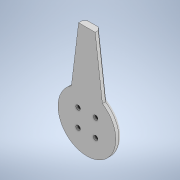
# Autodesk Inventor part: Pointerlever
Saved by Autodesk Inventor 2021 (Build 250183000, 183)
## iProperties
Created: 2024-04-28
Part Number: Pointerlever
Material: Generic
Document SubType Name: Modeling
Designer: Lukas
Density: 1 g/cm^3
Appearance: Default
Author: Lukas
Autodesk Inventor part; units mm, degrees
ref_plane "YZ Plane" through (0, 0, 0) normal (1, 0, 0) x (0, 1, 0)
ref_plane "XZ Plane" through (0, 0, 0) normal (0, 1, 0) x (-1, 0, 0)
ref_plane "XY Plane" through (0, 0, 0) normal (0, 0, 1) x (1, 0, 0)
sketch "Sketch1" plane through (0, 0, 0) normal (0, 0, 1) x (1, 0, 0)
  circle A0 centre (0, 0) radius 14
  circle A1 centre (-4.25, 4.25) radius 1.1
  circle A2 centre (-4.25, -4.25) radius 1.1
  circle A3 centre (4.25, -4.25) radius 1.1
  circle A4 centre (4.25, 4.25) radius 1.1
  line L0 (-7.5, 11.8216) -> (-4, 40)
  line L1 (-4, 40) -> (4, 40)
  line L2 (4, 40) -> (7.5, 11.8216)
  point P0 (0, 40)
  dimension "d0" = 8.5
  dimension "d1" = 8.5
  dimension "d2" = 4.25
  dimension "d3" = 4.25
  dimension "d4" = 2.2
  dimension "d5" = 28
  dimension "d6" = 8
  dimension "d7" = 15
  dimension "d8" = 40
  constraints: 6 end point, 5 centre point, 3 equal radius, 3 horizontal alignment, 3 vertical alignment, 2 point on circle, 1 coincident, 1 horizontal, 1 midpoint
  measures "d0" distance of A2.centre A1.centre
  measures "d1" distance of A3.centre A2.centre
  measures "d2" horizontal distance of point (0, 0) A2.centre
  measures "d3" horizontal distance of point (0, 0) A2.centre
  measures "d4" diameter of A1
  measures "d5" diameter of A0
  measures "d6" distance of L0.end L1.end
  measures "d7" distance of L2.end L0.start
  measures "d8" distance from line of point (0, 0) L1
extrude "Extrusion1" add sketch "Sketch1" along normal blind 1
sketch "Sketch2" plane through (0, 0, 0) normal (0, 0, 1) x (1, 0, 0)
  line L0 (7.5, 11.8216) -> (4, 40) projected
  line L1 (4, 40) -> (-4, 40) projected
  line L2 (-4, 40) -> (-7.5, 11.8216) projected
  arc A0 (-7.5, 11.8216) -> (7.5, 11.8216) centre (0, 0) ccw projected
  circle A1 centre (-4.25, 4.25) radius 1.1 projected
  circle A2 centre (-4.25, -4.25) radius 1.1 projected
  circle A3 centre (4.25, -4.25) radius 1.1 projected
  circle A4 centre (4.25, 4.25) radius 1.1 projected
  circle A5 centre (-4.25, 4.25) radius 2
  circle A6 centre (-4.25, -4.25) radius 1.1 projected
  circle A7 centre (-4.25, -4.25) radius 2
  circle A8 centre (4.25, -4.25) radius 1.1 projected
  circle A9 centre (4.25, -4.25) radius 2
  circle A10 centre (4.25, 4.25) radius 2
  dimension "d11" = 4
  constraints: 4 centre point, 4 coincident, 3 equal radius
  measures "d11" diameter of A5
extrude "Extrusion2" add sketch "Sketch2" against normal blind 2 contours A0 L2 L1 L0
chamfer "Chamfer1" distance 1.5 angle 45 2 edges at (-5.75, 25.9108, -2) (5.75, 25.9108, -2)
fillet "Fillet1" radius 1.5 1 edges at (0, -14, -2)
equation "\"d1\" = d0"
equation "\"d2\" = 0.5 * d1"
equation "\"d3\" = 0.5 * d0"
body "Solid1"
